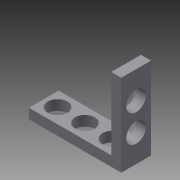
# Autodesk Inventor part: Equerre
Saved by Autodesk Inventor 2014 SP1 (Build 180222100, 222)
## iProperties
Created: 2014-04-23
Part Number: Equerre
Material: Generic
Document SubType Name: Modeling
Designer: david
Density: 1 g/cm^3
Appearance: Default
Author: david
Autodesk Inventor part; units mm, degrees
ref_plane "YZ Plane" through (0, 0, 0) normal (1, 0, 0) x (0, 1, 0)
ref_plane "XZ Plane" through (0, 0, 0) normal (0, 1, 0) x (-1, 0, 0)
ref_plane "XY Plane" through (0, 0, 0) normal (0, 0, 1) x (1, 0, 0)
sketch "Sketch1" plane through (0, 0, 0) normal (0, 1, 0) x (-1, 0, 0)
  line L0 (-10.1, 3.25) -> (10.1, 3.25)
  line L1 (10.1, 3.25) -> (10.1, -3.25)
  line L2 (10.1, -3.25) -> (-10.1, -3.25)
  line L3 (-10.1, -3.25) -> (-10.1, 3.25)
  line L4 (0, 0) -> (0, -7.2216) construction
  line L5 (0, 0) -> (18.1335, 0) construction
  dimension "d0" = 6.5
  dimension "d1" = 20.2
  constraints: 12 end point, 3 parallel, 2 perpendicular, 1 horizontal, 2 other
  measures "d0" distance between parallel lines of L2 L0
  measures "d1" distance between parallel lines of L1 L3
extrude "Extrusion1" add sketch "Sketch1" along normal blind 2.2
sketch "Sketch2" plane through (0, 2.2, 0) normal (0, 1, 0) x (1, 0, 0)
  line L0 (-10.1, -3.25) -> (10.1, -3.25) projected
  line L1 (10.1, -3.25) -> (10.1, 3.25) projected
  line L2 (10.1, 3.25) -> (-10.1, 3.25) projected
  line L3 (-10.1, 3.25) -> (-10.1, -3.25) projected
  line L4 (7.9, 3.25) -> (7.9, -3.25) construction
  line L5 (-1.1, 6.7296) -> (-1.1, -8.5112) construction
  circle A0 centre (-1.1, 0) radius 2.15
  circle A1 centre (-7.1, 0) radius 2.15
  circle A2 centre (4.9, 0) radius 2.15
  circle A3 centre (-1.1, 0) radius 2.15
  point P0 (0, 0)
  dimension "d4" = 2.2
  dimension "d5" = 4.3
  dimension "d8" = 6
  dimension "d11" = 6
  constraints: 4 centre point, 4 end point, 3 point on line, 2 horizontal, 1 parallel, 7 other
  measures "d4" distance between parallel lines of L1 L4
  measures "d5" diameter of A0
  measures "d8" distance of A0.centre A1.centre
  measures "d11" distance of A0.centre A2.centre
extrude "Extrusion2" cut sketch "Sketch2" against normal through all contours A0 | A1 | A2
sketch "Sketch3" plane through (0, 2.2, 0) normal (0, 1, 0) x (1, 0, 0)
  line L0 (10.1, 3.25) -> (-10.1, 3.25) projected
  line L1 (7.9, 3.25) -> (10.1, 3.25)
  line L2 (10.1, 3.25) -> (10.1, -3.25)
  line L3 (10.1, -3.25) -> (7.9, -3.25)
  line L4 (7.9, -3.25) -> (7.9, 3.25)
  point P0 (0, 0)
  dimension "d19" = 2.2
  constraints: 8 end point, 2 parallel, 1 horizontal, 1 perpendicular, 1 point on line
  measures "d19" distance between parallel lines of L2 L4
extrude "Extrusion3" add sketch "Sketch3" along normal blind 15.8
sketch "Sketch4" plane through (10.1, 0, 3.25) normal (1, 0, 0) x (0, 0, -1)
  line L0 (0, 0) -> (0, 18) projected
  line L1 (3.25, 19.7577) -> (3.25, -0.3358) construction
  circle A0 centre (3.25, 6) radius 2.15
  circle A1 centre (3.25, 12) radius 2.15
  point P0 (3.25, 0)
  dimension "d22" = 4.3
  dimension "d23" = 4.3
  dimension "d24" = 6
  dimension "d25" = 6
  constraints: 2 centre point, 2 end point, 2 point on line, 1 parallel
  measures "d22" diameter of A1
  measures "d23" diameter of A0
  measures "d24" distance of point (3.25, 0) A0.centre
  measures "d25" distance of A0.centre A1.centre
extrude "Extrusion4" cut sketch "Sketch4" against normal through all
equation "\"d2\" = Depth"
equation "\"d4\" = Depth"
equation "\"d5\" = Holes"
equation "\"d17\" = Depth"
equation "\"d19\" = Depth"
equation "\"d22\" = Holes"
equation "\"d23\" = Holes"
equation "\"Holes\" = 4.3"
equation "\"Depth\" = 2.2"
body "Solid1"
